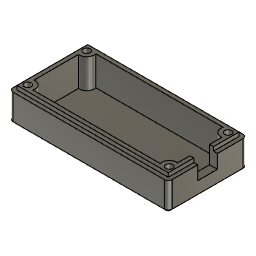
MG996R_Shell_Bottom v2 (Autodesk Fusion 360 design; units mm, degrees)
Autodesk Fusion 360 part; units mm, degrees
sketch "Sketch1" plane through (0, 0, 0) normal (0, 0, 1) x (1, 0, 0)
  line L0 (20.25, 10) -> (-20.25, 10)
  line L1 (-20.25, 10) -> (-20.25, -10)
  line L2 (-20.25, -10) -> (20.25, -10)
  line L3 (20.25, -10) -> (20.25, 10)
  line L4 (20.25, 10) -> (-20.25, -10) construction
  line L5 (-20.25, 10) -> (20.25, -10) construction
  dimension "d1" = 40.5
  dimension "d2" = 20
  constraint horizontal L0
  constraint perpendicular L0 L1
  constraint parallel L0 L2
  constraint parallel L1 L3
  constraint coincident L4 origin
  constraint coincident L5 origin
  measures "d1" distance of L0.start L0.end
  measures "d2" distance of L0.start L2.end
extrude "Extrude1" add sketch "Sketch1" along normal blind 8.53
sketch "Sketch2" plane through (0, 0, 8.53) normal (0, 0, 1) x (-1, 0, 0)
  line L0 (-20.25, 10) -> (-20.25, -10)
  line L1 (-20.25, -10) -> (20.25, -10)
  line L2 (20.25, -10) -> (20.25, 10)
  line L3 (20.25, 10) -> (-20.25, 10)
  line L4 (-18, -7.5) -> (18, -7.5) construction
  line L5 (18, -7.5) -> (18, 7.5) construction
  line L6 (18, 7.5) -> (-18, 7.5) construction
  line L7 (-18, 7.5) -> (-18, -7.5) construction
  line L8 (-18, -7.5) -> (18, 7.5) construction
  line L9 (18, -7.5) -> (-18, 7.5) construction
  circle A0 centre (-18, -7.5) radius 0.875
  circle A1 centre (-18, 7.5) radius 0.875
  circle A2 centre (18, 7.5) radius 0.875
  circle A3 centre (18, -7.5) radius 0.875
  dimension "d6" = 15
  dimension "d7" = 36
  dimension "d8" = 1.75
  constraint horizontal L4
  constraint perpendicular L4 L5
  constraint parallel L4 L6
  constraint parallel L5 L7
  constraint coincident L8 origin
  constraint coincident L9 origin
  constraint coincident L4.start L7.end
  constraint coincident L6.end L7.start
  constraint coincident L5.end L6.start
  constraint coincident L4.end L5.start
  constraint equal A2 A3
  constraint equal A0 A2
  constraint equal A0 A1
  measures "d6" distance of L4.end L5.end
  measures "d7" distance of L4.start L4.end
  measures "d8" diameter of A3
extrude "Extrude2" cut sketch "Sketch2" against normal blind 15 contours A0 | A1 | A2 | A3
sketch "Sketch3" plane through (0, 0, 8.53) normal (0, 0, 1) x (-1, 0, 0)
  circle A0 centre (-18, -7.5) radius 0.875
  circle A1 centre (-18, 7.5) radius 0.875
  circle A2 centre (18, -7.5) radius 0.875
  circle A3 centre (18, 7.5) radius 0.875
  line L0 (-20.25, 10) -> (-20.25, -10)
  line L1 (-20.25, -10) -> (20.25, -10)
  line L2 (20.25, -10) -> (20.25, 10)
  line L3 (20.25, 10) -> (-20.25, 10)
  line L4 (-18.25, -8) -> (18.25, -8)
  line L5 (18.25, -8) -> (18.25, 8)
  line L6 (18.25, 8) -> (-18.25, 8)
  line L7 (-18.25, 8) -> (-18.25, -8)
  line L8 (-18.25, -8) -> (18.25, 8) construction
  line L9 (18.25, -8) -> (-18.25, 8) construction
  circle A4 centre (-18, -7.5) radius 1.875
  circle A5 centre (-18, 7.5) radius 1.875
  circle A6 centre (18, 7.5) radius 1.875
  circle A7 centre (18, -7.5) radius 1.875
  dimension "d11" = 2
  dimension "d13" = 2
  dimension "d14" = 3.75
  constraint horizontal L4
  constraint perpendicular L4 L5
  constraint parallel L4 L6
  constraint parallel L5 L7
  constraint coincident L8 origin
  constraint coincident L9 origin
  constraint concentric A0 A4
  constraint concentric A1 A5
  constraint concentric A3 A6
  constraint concentric A2 A7
  constraint equal A6 A7
  constraint equal A5 A6
  constraint equal A4 A5
  measures "d11" distance of L1 L4
  measures "d13" distance of L0 L7
  measures "d14" diameter of A7
extrude "Extrude3" cut sketch "Sketch3" against normal blind 7.5 contours L4 L5 L6 L7 A4 A5 A6 A7
sketch "Sketch4" plane through (20.25, 0, 0) normal (1, 0, 0) x (0, 1, 0)
  line L0 (-10, 0) -> (10, 0)
  line L1 (10, 0) -> (10, 8.53)
  line L2 (10, 8.53) -> (-10, 8.53)
  line L3 (-10, 8.53) -> (-10, 0)
  line L4 (-2.5, 8.53) -> (2.5, 8.53)
  line L5 (2.5, 8.53) -> (2.5, 4.03)
  line L6 (2.5, 4.03) -> (-2.5, 4.03)
  line L7 (-2.5, 4.03) -> (-2.5, 8.53)
  dimension "d17" = 5
  dimension "d18" = 4.5
  dimension "d19" = 2.5
  constraint horizontal L4
  constraint vertical L5
  constraint horizontal L6
  constraint vertical L7
  constraint coincident L2 L4.start
  measures "d17" distance of L4.start L4.end
  measures "d18" distance of L4.start L6.end
  measures "d19" distance of origin L7
extrude "Extrude4" cut sketch "Sketch4" against normal blind 3 contours L2 L4 L5 L6 L7
sketch "Sketch5" plane through (0, 0, 8.53) normal (0, 0, 1) x (-1, 0, 0)
  line L0 (-20.25, 2.5) -> (-18.25, 2.5)
  line L1 (-18.25, 2.5) -> (-18.25, 5.6417)
  arc A0 (-18.25, 5.6417) -> (-16.1929, 8) centre (-18, 7.5) ccw
  line L2 (-16.1929, 8) -> (16.1929, 8)
  arc A1 (16.1929, 8) -> (18.25, 5.6417) centre (18, 7.5) ccw
  line L3 (18.25, 5.6417) -> (18.25, -5.6417)
  arc A2 (18.25, -5.6417) -> (16.1929, -8) centre (18, -7.5) ccw
  line L4 (16.1929, -8) -> (-16.1929, -8)
  arc A3 (-16.1929, -8) -> (-18.25, -5.6417) centre (-18, -7.5) ccw
  line L5 (-18.25, -5.6417) -> (-18.25, -2.5)
  line L6 (-18.25, -2.5) -> (-20.25, -2.5)
  line L7 (-20.25, -2.5) -> (-20.25, -10)
  line L8 (-20.25, -10) -> (20.25, -10)
  line L9 (20.25, -10) -> (20.25, 10)
  line L10 (20.25, 10) -> (-20.25, 10)
  line L11 (-20.25, 10) -> (-20.25, 2.5)
  circle A4 centre (-18, -7.5) radius 0.875
  circle A5 centre (-18, 7.5) radius 0.875
  circle A6 centre (18, -7.5) radius 0.875
  circle A7 centre (18, 7.5) radius 0.875
  line L12 (19.25, -9) -> (-19.25, -9)
  line L13 (-19.25, -9) -> (-19.25, 9)
  line L14 (-19.25, 9) -> (19.25, 9)
  line L15 (19.25, 9) -> (19.25, -9)
  line L16 (19.25, -9) -> (-19.25, 9) construction
  line L17 (-19.25, -9) -> (19.25, 9) construction
  dimension "d22" = 1
  dimension "d23" = 1
  constraint horizontal L12
  constraint perpendicular L12 L13
  constraint parallel L12 L14
  constraint parallel L13 L15
  constraint coincident L16 origin
  constraint coincident L17 origin
  measures "d22" distance of L8 L12
  measures "d23" distance of L9 L15
extrude "Extrude5" cut sketch "Sketch5" against normal blind 1 contours L0 L6 L7 L8 L9 L10 L11 L12 L13 L14 L15
fillet "Fillet1" radius 1 4 edges at (-20.25, -10, 3.765) (-20.25, 10, 3.765) (20.25, -10, 3.765) (20.25, 10, 3.765)
chamfer "Chamfer1" distance 1 angle 45 8 edges at (0, 10, 0) (-19.9571, 9.7071, 0) (-20.25, 0, 0) (-19.9571, -9.7071, 0) (0, -10, 0) (19.9571, -9.7071, 0) (20.25, 0, 0) (19.9571, 9.7071, 0)
sketch "Sketch6" plane through (0, 0, 0) normal (0, 0, -1) x (1, 0, 0)
  circle A0 centre (-18, 7.5) radius 0.875
  circle A1 centre (-18, -7.5) radius 0.875
  circle A2 centre (18, 7.5) radius 0.875
  circle A3 centre (18, -7.5) radius 0.875
  line L0 (-19.25, -9) -> (19.25, -9)
  line L1 (19.25, -9) -> (19.25, 9)
  line L2 (19.25, 9) -> (-19.25, 9)
  line L3 (-19.25, 9) -> (-19.25, -9)
  circle A4 centre (-19.25, 9) radius 5
  circle A5 centre (19.25, 9) radius 5
  circle A6 centre (19.25, -9) radius 5
  circle A7 centre (-19.25, -9) radius 5
  dimension "d29" = 10
  constraint equal A4 A7
  constraint equal A4 A5
  constraint equal A5 A6
  constraint coincident L2.end L3.start
  constraint coincident L0.start L3.end
  constraint coincident L1.end L2.start
  constraint coincident L0.end L1.start
  measures "d29" diameter of A4
extrude "Extrude6" cut sketch "Sketch6" against normal blind 0.5 contours L0 L3 A7 | L0 L3 A7 | L0 L1 A6 | L0 L1 A6 | L2 L3 A4 | L2 L3 A4 | L1 L2 A5 | L1 L2 A5
